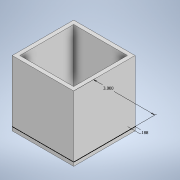
# Autodesk Inventor part: squareMouseSupport
Saved by Autodesk Inventor 2022 (Build 260153000, 153)
## iProperties
Created: 2021-04-17
Part Number: squareMouseSupport
Material: Generic
Document SubType Name: Modeling
Designer: robst
Density: 1 g/cm^3
Appearance: Default
Author: robst
Autodesk Inventor part; units mm, degrees
ref_plane "YZ Plane" through (0, 0, 0) normal (1, 0, 0) x (0, 1, 0)
ref_plane "XZ Plane" through (0, 0, 0) normal (0, 1, 0) x (-1, 0, 0)
ref_plane "XY Plane" through (0, 0, 0) normal (0, 0, 1) x (1, 0, 0)
sketch "Sketch1" plane through (0, 0, 0) normal (0, 1, 0) x (-1, 0, 0)
  line L0 (-38.1, 38.1) -> (-38.1, -38.1)
  line L1 (-38.1, -38.1) -> (38.1, -38.1)
  line L2 (38.1, -38.1) -> (38.1, 38.1)
  line L3 (38.1, 38.1) -> (-38.1, 38.1)
  line L4 (-38.1, 38.1) -> (38.1, -38.1) construction
  line L5 (-38.1, -38.1) -> (38.1, 38.1) construction
  line L6 (-33.3375, 33.3375) -> (-33.3375, -33.3375)
  line L7 (-33.3375, -33.3375) -> (33.3375, -33.3375)
  line L8 (33.3375, -33.3375) -> (33.3375, 33.3375)
  line L9 (33.3375, 33.3375) -> (-33.3375, 33.3375)
  line L10 (-33.3375, 33.3375) -> (33.3375, -33.3375) construction
  line L11 (-33.3375, -33.3375) -> (33.3375, 33.3375) construction
  point P0 (0, 0)
  dimension "d0" = 76.2
  dimension "d1" = 4.7625
  constraints: 24 end point, 4 midpoint, 4 parallel, 4 perpendicular, 2 vertical
  measures "d0" distance of L0.end L1.end
  measures "d1" distance between parallel lines of L7 L1
extrude "Extrusion1" add sketch "Sketch1" against normal blind 4.7625 contours L3 L2 L1 L0 | L9 L8 L7 L6
extrude "Extrusion2" add sketch "Sketch1" along normal blind 76.2
body "Solid1"
